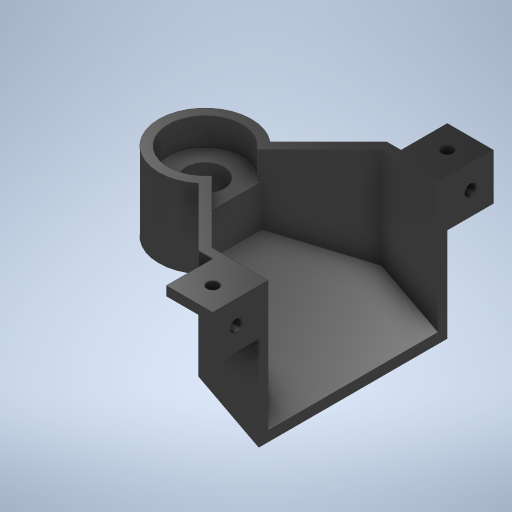
# Autodesk Inventor part: Rampa2
Saved by Autodesk Inventor 2023 (Build 270158000, 158)
## iProperties
Created: 2022-12-03
Part Number: Rampa2
Material: Genérico
Document SubType Name: Modeling
Designer: sergi
Density: 1 g/cm^3
Appearance: Valor por defecto
Author: sergi
Autodesk Inventor part; units mm, degrees
ref_plane "YZ Plane" through (0, 0, 0) normal (1, 0, 0) x (0, 1, 0)
ref_plane "XZ Plane" through (0, 0, 0) normal (0, 1, 0) x (-1, 0, 0)
ref_plane "XY Plane" through (0, 0, 0) normal (0, 0, 1) x (1, 0, 0)
sketch "Boceto1" plane through (0, 0, 0) normal (0, 1, 0) x (-1, 0, 0)
  circle A0 centre (0, 0) radius 4.1
  arc A1 (-6.3308, -7.7408) -> (-6.3308, 7.7408) centre (0, 0) ccw
  line L0 (-18.96, -20.37) -> (-32, -20.37)
  line L1 (-32, -20.37) -> (-32, 20.37)
  line L2 (-32, 20.37) -> (-18.96, 20.37)
  line L3 (-18.96, 20.37) -> (-6.3308, 7.7408)
  line L4 (-18.96, -20.37) -> (-6.3308, -7.7408)
  dimension "d15" = 13.04
  dimension "d16" = 40.74
  dimension "d17" = 13.04
  constraints: 10 end point, 3 perpendicular, 2 centre point, 2 point on circle, 1 horizontal
  measures "d15" distance of L0.start L0.end
  measures "d16" distance of L0.end L1.end
  measures "d17" distance of L1.end L2.end
extrude "Extrusión1" add sketch "Boceto1" along normal blind 20.31
sketch "Boceto2" plane through (0, 0, 0) normal (0, -1, 0) x (1, 0, 0)
  arc A0 (6.3308, 7.7408) -> (6.3308, -7.7408) centre (0, 0) ccw projected
  arc A1 (6.3308, 7.7408) -> (6.3308, -7.7408) centre (0, 0) ccw projected
  line L0 (6.3308, -7.7408) -> (6.3308, 7.7408)
  constraints: 2 end point
extrude "Extrusión2" cut sketch "Boceto2" against normal blind 13.31
chamfer "Chaflán1" distance 13.31 angle 62.5 1 edges at (6.3308, 0, 0) measured on face at (6.3308, 0.5, 0)
shell "Vaciado1" thickness 2 removed faces 3 at (23.4436, 20.31, -2.5803) at (32, 6.77, 6.79) at (-4.0469, 15.6433, 0.6577)
sketch "Boceto7" plane through (0, 20.31, 0) normal (0, 1, 0) x (1, 0, 0)
  line L0 (6.8202, -5.4018) -> (6.8202, 5.4018) projected
  line L1 (19.7884, 18.37) -> (32, 18.37) projected
  line L2 (32, 18.37) -> (32, 20.37) projected
  line L3 (32, 20.37) -> (18.96, 20.37) projected
  line L4 (18.96, 20.37) -> (6.3308, 7.7408) projected
  arc A0 (6.3308, 7.7408) -> (6.3308, -7.7408) centre (0, 0) ccw projected
  line L5 (6.3308, -7.7408) -> (18.96, -20.37) projected
  line L6 (18.96, -20.37) -> (32, -20.37) projected
  line L7 (32, -20.37) -> (32, -18.37) projected
  line L8 (32, -18.37) -> (19.7884, -18.37) projected
  line L9 (19.7884, -18.37) -> (6.3214, -4.903) projected
  arc A1 (6.3214, 4.903) -> (6.3214, -4.903) centre (0, 0) ccw projected
  line L10 (6.3214, 4.903) -> (19.7884, 18.37) projected
extrude "Extrusión5" add sketch "Boceto7" along normal blind 10 contours L9 L8 L7 L6 L5 A0 L4 L3 L2 L1 L10 A1
sketch "Boceto8" plane through (18.96, 30.31, 20.37) normal (0, 0, 1) x (1, 0, 0)
  line L0 (13.04, 0) -> (0.8284, 0) projected
  line L1 (13.04, 0) -> (11.04, 0)
  line L2 (11.04, 0) -> (11.04, -10)
  line L3 (11.04, -10) -> (13.04, -10)
  line L4 (13.04, -10) -> (13.04, 0)
  line L5 (13.04, 0) -> (3.04, 0)
  line L6 (3.04, 0) -> (3.04, -2)
  line L7 (3.04, -2) -> (13.04, -2)
  line L8 (13.04, -2) -> (13.04, 0)
  point P0 (-18.96, -30.31)
  point P1 (11.04, -2)
  dimension "d72" = 2
  dimension "d73" = 10
  dimension "d74" = 10
  dimension "d75" = 2
  constraints: 16 end point, 4 parallel, 2 horizontal, 2 perpendicular
  measures "d72" distance of L3.end L2.end
  measures "d73" distance of L2.end L1.end
  measures "d74" distance of L7.end L6.end
  measures "d75" distance of L6.end L5.end
extrude "Extrusión6" add sketch "Boceto8" along normal blind 10
sketch "Boceto11" plane through (32, 30.31, -20.37) normal (0, 0, -1) x (-1, 0, 0)
  line L0 (0, 0) -> (10, 0)
  line L1 (10, 0) -> (10, -2)
  line L2 (10, -2) -> (0, -2)
  line L3 (0, -2) -> (0, 0)
  line L4 (0, 0) -> (2, 0)
  line L5 (2, 0) -> (2, -10)
  line L6 (2, -10) -> (0, -10)
  line L7 (0, -10) -> (0, 0)
  point P0 (32, -30.31)
  point P1 (2, -2)
  point P2 (0, -2)
  dimension "d96" = 10
  dimension "d97" = 2
  dimension "d98" = 2
  dimension "d99" = 10
  constraints: 16 end point, 4 parallel, 2 horizontal, 2 perpendicular
  measures "d96" distance of L1.end L2.end
  measures "d97" distance of L0.end L1.end
  measures "d98" distance of L5.end L6.end
  measures "d99" distance of L4.end L5.end
extrude "Extrusión7" add sketch "Boceto11" along normal blind 10
sketch "Boceto9" plane through (32, 0, 20.37) normal (1, 0, 0) x (0, 0, -1)
  line L0 (-10, 20.31) -> (-10, 30.31) projected
  line L1 (2, 30.31) -> (-10, 30.31) projected
  line L2 (50.74, 30.31) -> (50.74, 20.31) projected
  line L3 (40.74, 20.31) -> (50.74, 20.31) projected
  point P0 (20.37, 0)
  point P1 (-5, 25.31)
  point P2 (45.74, 25.31)
  dimension "d78" = 5
  dimension "d79" = 5
  dimension "d102" = 5
  dimension "d103" = 5
  measures "d78" distance from line of L0 point (-5, 25.31)
  measures "d79" distance from line of L1 point (-5, 25.31)
  measures "d102" distance from line of L2 point (45.74, 25.31)
  measures "d103" distance from line of L3 point (45.74, 25.31)
hole "Agujero3" at (32, 25.31, 25.37) at (32, 25.31, -25.37) direction (-1, 0, 0) diameter 2.5 depth 8
sketch "Boceto10" plane through (0, 30.31, 0) normal (0, 1, 0) x (1, 0, 0)
  line L0 (32, -30.37) -> (22, -30.37) projected
  line L1 (22, -20.37) -> (22, -30.37) projected
  line L2 (22, 30.37) -> (32, 30.37) projected
  line L3 (22, 20.37) -> (22, 30.37) projected
  point P0 (0, 0)
  point P1 (27, -25.37)
  point P2 (27, 25.37)
  dimension "d87" = 5
  dimension "d88" = 5
  dimension "d104" = 5
  dimension "d105" = 5
  measures "d87" distance from line of L0 point (27, -25.37)
  measures "d88" distance from line of L1 point (27, -25.37)
  measures "d104" distance from line of L2 point (27, 25.37)
  measures "d105" distance from line of L3 point (27, 25.37)
hole "Agujero4" at (27, 30.31, 25.37) at (27, 30.31, -25.37) direction (0, -1, 0) diameter 2.5 depth 8
sketch "Boceto12" plane through (0, 15.31, 0) normal (0, 1, 0) x (1, 0, 0)
  circle A0 centre (0, 0) radius 4.1 projected
  arc A1 (6.3214, 4.903) -> (6.3214, -4.903) centre (0, 0) ccw projected
  line L0 (6.8202, -5.4018) -> (6.3214, -4.903) projected
  line L1 (6.8202, -5.4018) -> (6.8202, 5.4018) projected
  line L2 (6.3214, 4.903) -> (6.8202, 5.4018) projected
extrude "Extrusión8" add sketch "Boceto12" along normal blind 9
